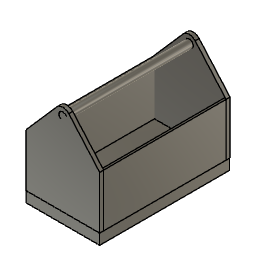
first 3d work v3 (Autodesk Fusion 360 design; units mm, degrees)
Autodesk Fusion 360 part; units mm, degrees
sketch "Sketch1" plane through (0, 0, 0) normal (0, 1, 0) x (1, 0, 0) in component "Component"
  line L0 (0, 0) -> (0, -12)
  line L1 (0, -12) -> (14, -12)
  line L2 (14, -12) -> (14, 0)
  line L3 (14, 0) -> (0, 0)
  line L4 (5.8711, -18.7099) -> (0, -12)
  line L5 (8.1289, -18.7099) -> (14, -12)
  arc A0 (5.8711, -18.7099) -> (8.1289, -18.7099) centre (7, -17.7221) ccw
  circle A1 centre (7, -17.7221) radius 0.75
  dimension "d2" = 1.5
  constraint coincident L0.start L3.end
  constraint vertical L0
  constraint perpendicular L0 L1
  constraint perpendicular L1 L2
  constraint perpendicular L2 L3
  measures "d2" radius of A0
extrude "Extrude1" add sketch "Sketch1" along normal blind 0.75 makes body 1 in component "Component"
sketch "Sketch2" plane through (0, 0.75, 0) normal (0, 1, 0) x (-1, 0, 0) in component "Component"
  circle A0 centre (-7, 17.7221) radius 0.75
  arc A1 (-5.8711, 18.7099) -> (-8.1289, 18.7099) centre (-7, 17.7221) ccw
  line L0 (-8.1289, 18.7099) -> (-14, 12)
  line L1 (-14, 12) -> (-14, 0)
  line L2 (-14, 0) -> (0, 0)
  line L3 (0, 0) -> (0, 12)
  line L4 (0, 12) -> (-5.8711, 18.7099)
  line L5 (-14, 0) -> (-13.6, 0)
  line L6 (-14, 12) -> (-13.6, 12)
  line L7 (-13.6, 12) -> (-13.6, 0)
  constraint coincident L1.end L2.start
  constraint coincident L2 L5.end
  constraint perpendicular L1 L5
  constraint coincident L0.end L1.start
  constraint perpendicular L1 L6
  constraint perpendicular L2 L7
extrude "Extrude2" add sketch "Sketch2" along normal blind 24 separate body contours L1 L2 L5 L6 L7 makes body 2 in component "Component"
copy_body "CopyPasteBodies1" bodies 2 makes body 3 in component "Component"
move_body "Move1" bodies 3 to x (1, 0, 0) y (0, 1, 0) z (0, 0, 1) at (0, 0, 0) in component "Component"
copy_body "CopyPasteBodies2" bodies 2 makes body 4 in component "Component"
move_body "Move2" bodies 4 to x (1, 0, 0) y (0, 1, 0) z (0, 0, 1) at (0, 0, 0) in component "Component"
copy_body "CopyPasteBodies3" bodies 3 makes body 5 in component "Component"
move_body "Move3" bodies 5 to x (1, 0, 0) y (0, 1, 0) z (0, 0, 1) at (-13.6, 0, 0) in component "Component"
copy_body "CopyPasteBodies4" bodies 1 makes body 6 in component "Component"
move_body "Move4" bodies 6 to x (1, 0, 0) y (0, 1, 0) z (0, 0, 1) at (0, 24, 0) in component "Component"
sketch "Sketch3" plane through (0, 24.75, 0) normal (0, 1, 0) x (-1, 0, 0) in component "Component"
  line L0 (-14, 12) -> (-14, 0)
  line L1 (-14, 0) -> (-13.6, 0)
  line L2 (-13.6, 0) -> (-13.6, 12)
  line L3 (-13.6, 12) -> (-14, 12)
  line L4 (-13.6136, 0, -24) -> (0.4769, 0, -24)
  line L5 (0.4769, 0, -24) -> (0.4769, 39.4927, -24)
  line L6 (0.4769, 39.4927, -24) -> (-13.6136, 39.4927, -24)
  line L7 (-13.6136, 39.4927, -24) -> (-13.6136, 0, -24)
  line L8 (0, 0) -> (-16, 0)
  line L9 (-16, 0) -> (-16, -42)
  line L10 (-16, -42) -> (0, -42)
  line L11 (0, -42) -> (0, 0)
  constraint horizontal L8
  constraint vertical L9
  constraint horizontal L10
  constraint vertical L11
sketch "Sketch4" plane through (0, 0, 0) normal (0, 0, 1) x (1, 0, 0) in component "Component"
  line L0 (14, 25) -> (0, 25)
  line L1 (0, 25) -> (0, 0)
  line L2 (0, 0) -> (14, 0)
  line L3 (14, 0) -> (14, 25)
  constraint horizontal L0
  constraint vertical L1
  constraint horizontal L2
  constraint vertical L3
  constraint coincident L1.end L2.start
extrude "Extrude4" cut sketch "Sketch4" along normal blind 2 bodies 1 2 3 4 5 6 in component "Component"
sketch "Sketch5" plane through (0, 0, 0) normal (0, 0, 1) x (1, 0, 0) in component "Component"
  line L0 (14, 0) -> (0.0352, 0)
  line L1 (0.0352, 0) -> (0.0352, 24.6816)
  line L2 (0.0352, 24.6816) -> (14, 24.6816)
  line L3 (14, 24.6816) -> (14, 0)
  constraint horizontal L0
  constraint vertical L1
  constraint horizontal L2
  constraint vertical L3
extrude "Extrude5" add sketch "Sketch5" along normal blind 2 separate body makes body 7 in component "Component"
sketch "Sketch6" plane through (0, 0, 0) normal (0, 1, 0) x (1, 0, 0) in component "Component"
  circle A0 centre (7.027, -17.6921) radius 0.7418
extrude "Extrude6" add sketch "Sketch6" along normal blind 24 bodies 1 7 6 in component "Component"
move_face "MoveFace1" to x (1, 0, 0) y (0, 1, 0) z (0, 0, 1) at (-20.5818, 1, -7.5096) 1 faces at (6.6026, 8.5, 17.0838) on bodies 1 in component "Component"
component "Component" placed x (1, 0, 0) y (0, 1, 0) z (0, 0, 1) at (0, 0, 0)
equation "d4 = ( 3 / 4 ) * 1 mm"
